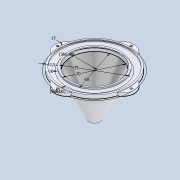
# Autodesk Inventor part: LilghtPointLensHolder
Saved by Autodesk Inventor 2020.3 (Build 243373010, 373A)
## iProperties
Created: 2020-12-04
Part Number: LilghtPointLensHolder
Material: Generic
Document SubType Name: Modeling
Designer: Yusuf
Mass: 40.7288 g
Surface Area: 309.662 cm^2
Volume: 40.7288 cm^3
Density: 1 g/cm^3
Appearance: Default
Author: Yusuf
Autodesk Inventor part; units mm, degrees
ref_plane "YZ Plane" through (0, 0, 0) normal (1, 0, 0) x (0, 1, 0)
ref_plane "XZ Plane" through (0, 0, 0) normal (0, 1, 0) x (-1, 0, 0)
ref_plane "XY Plane" through (0, 0, 0) normal (0, 0, 1) x (1, 0, 0)
sketch "Sketch1" plane through (0, 0, 0) normal (0, 1, 0) x (-1, 0, 0)
  circle A0 centre (0, 0) radius 35
  circle A1 centre (0, 0) radius 34
  circle A2 centre (0, 0) radius 37.5
  circle A3 centre (0, 0) radius 50
  circle A4 centre (0, 0) radius 47.5
  arc A5 (47.6375, -15.1878) -> (47.6375, 15.1878) centre (40, 0) ccw
  arc A6 (15.1878, 47.6375) -> (-15.1878, 47.6375) centre (0, 40) ccw
  arc A7 (-47.6375, 15.1878) -> (-47.6375, -15.1878) centre (-40, 0) ccw
  arc A8 (-15.1878, -47.6375) -> (15.1878, -47.6375) centre (0, -40) ccw
  point P0 (-15.1878, -47.6375)
  point P1 (-47.6375, -15.1878)
  point P2 (-47.6375, 15.1878)
  point P3 (-15.1878, 47.6375)
  point P4 (0, 53)
  point P5 (-53, 0)
  point P6 (-40, 0)
  point P7 (0, -53)
  point P8 (53, 0)
  point P9 (40, 0)
  dimension "d6" = 70
  dimension "d7" = 68
  dimension "d8" = 75
  dimension "d11" = 10
  dimension "d12" = 2.5
  dimension "d13" = 17
  dimension "d14" = 40
  dimension "d17" = 360
  dimension "d27" = 13
  dimension "d30" = 360
  constraints: 10 point on circle, 9 centre point, 5 coincident, 2 vertical alignment, 26 other
  measures "d6" diameter of A0
  measures "d7" diameter of A1
  measures "d8" diameter of A2
  measures "d11" radial gap between concentric circles of A4 A2
  measures "d12" radial gap between concentric circles of A4 A3
  measures "d13" radius of A5
  measures "d14" distance of A2.centre A5.centre
  measures "d27" distance of point (0, 53) A6.centre
extrude "Extrusion1" add sketch "Sketch1" along normal blind 5 contours A2 | A3
extrude "Extrusion2" add sketch "Sketch1" along normal blind 3 contours A4
extrude "Extrusion3" add sketch "Sketch1" along normal blind 4 contours A3 A5 | A3 A6 | A8 A3 | A3 A7
extrude "Extrusion4" add sketch "Sketch1" along normal blind 4 contours A0
hole "Hole1" at (0, 0, 53) at (53, 0, 0) at (0, 0, -53) at (-53, 0, 0) direction (0, 1, 0) diameter 3.242 depth 11.8 thread size "M4x0.7" class "6H" standard "ANSI Metric M Profile"
sketch "Sketch2" plane through (0, 0, 0) normal (1, 0, 0) x (0, 1, 0)
  line L0 (0, 0) -> (0, 34)
  line L1 (0, 15.1878) -> (0, 47.6375) projected
  line L2 (0, 34) -> (0, 35)
  line L3 (0, 35) -> (-60, 35)
  line L4 (-60, 35) -> (-60, 5)
  line L5 (-60, 5) -> (0, 34)
  line L6 (-60, 8) -> (-4.1379, 35)
  line L7 (-4.1379, 35) -> (0, 37)
  line L8 (-72, 0) -> (12, 0) projected
  dimension "d39" = 34
  dimension "d40" = 1
  dimension "d41" = 60
  dimension "d42" = 30
  dimension "d43" = 3
  dimension "d44" = 3
  constraints: 14 end point, 5 point on line, 1 horizontal, 1 parallel, 1 perpendicular
  measures "d39" distance of L0.start L0.end
  measures "d40" distance of L0.end L2.end
  measures "d41" distance of L2.end L3.end
  measures "d42" distance of L3.end L4.end
  measures "d43" distance of L4.end L6.start
  measures "d44" distance of L0.end L7.end
revolve "Revolution1" add sketch "Sketch2" angle 360 about axis through (0, -10, 0) along (0, 1, 0) contours L5 L4 L6 L3 L1
body "Solid1"
